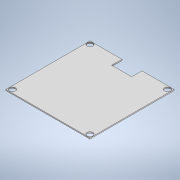
# Autodesk Inventor part: Bottom Cover
Saved by Autodesk Inventor 2020 (Build 240168000, 168)
## iProperties
Created: 2019-07-24
Part Number: Bottom Cover
Material: Generic
Document SubType Name: Modeling
Designer: Paul
Density: 1 g/cm^3
Appearance: Default
Author: Paul
Autodesk Inventor part; units mm, degrees
ref_plane "YZ Plane" through (0, 0, 0) normal (1, 0, 0) x (0, 1, 0)
ref_plane "XZ Plane" through (0, 0, 0) normal (0, 1, 0) x (-1, 0, 0)
ref_plane "XY Plane" through (0, 0, 0) normal (0, 0, 1) x (1, 0, 0)
sketch "Sketch1" plane through (0, 0, 0) normal (0, 1, 0) x (-1, 0, 0)
  line L0 (16, 16) -> (-16, 16)
  line L1 (-16, 16) -> (-16, -16)
  line L2 (-16, -16) -> (16, -16)
  line L3 (16, -16) -> (16, 16)
  line L4 (16, 16) -> (-16, -16) construction
  line L5 (-16, 16) -> (16, -16) construction
  point P0 (0, 0)
  dimension "d0" = 32
  dimension "d1" = 32
  constraints: 12 end point, 2 midpoint, 2 parallel, 1 horizontal, 1 perpendicular
  measures "d0" distance of L2.end L1.end
  measures "d1" distance of L1.end L0.end
extrude "Extrusion1" add sketch "Sketch1" along normal blind 0.4
sketch "Sketch2" plane through (0, 0.4, 0) normal (0, 1, 0) x (1, 0, 0)
  circle A0 centre (-14.76, -14.76) radius 1.11
  circle A1 centre (-14.76, 14.76) radius 1.11
  circle A2 centre (14.76, 14.76) radius 1.11
  circle A3 centre (14.76, -14.76) radius 1.11
  line L0 (16, 16) -> (-16, 16) projected
  line L1 (-16, 16) -> (-16, -16) projected
  line L2 (16, -16) -> (16, 16) projected
  line L3 (-16, -16) -> (16, -16) projected
  point P0 (0, 0)
  dimension "d16" = 2.22
  dimension "d17" = 2.22
  dimension "d18" = 2.22
  dimension "d19" = 2.22
  dimension "d20" = 1.24
  dimension "d21" = 1.24
  dimension "d22" = 1.24
  dimension "d23" = 1.24
  dimension "d24" = 1.24
  dimension "d25" = 1.24
  dimension "d26" = 1.24
  dimension "d27" = 1.24
  constraints: 4 centre point
  measures "d16" diameter of A0
  measures "d17" diameter of A1
  measures "d18" diameter of A2
  measures "d19" diameter of A3
  measures "d20" distance from line of L0 A1.centre
  measures "d21" distance from line of L1 A1.centre
  measures "d22" distance from line of L0 A2.centre
  measures "d23" distance from line of L2 A2.centre
  measures "d24" distance from line of L2 A3.centre
  measures "d25" distance from line of L3 A3.centre
  measures "d26" distance from line of L1 A0.centre
  measures "d27" distance from line of L3 A0.centre
extrude "Extrusion2" cut sketch "Sketch2" against normal blind 0.4 contours A0 | A1 | A2 | A3
sketch "Sketch3" plane through (0, 0.4, 0) normal (0, 1, 0) x (1, 0, 0)
  line L0 (-3.8, 16) -> (3.8, 16)
  line L1 (3.8, 16) -> (3.8, 12.1)
  line L2 (3.8, 12.1) -> (-3.8, 12.1)
  line L3 (-3.8, 12.1) -> (-3.8, 16)
  line L4 (16, 16) -> (-16, 16) projected
  line L5 (16, -16) -> (16, 16) projected
  dimension "d32" = 7.6
  dimension "d33" = 3.9
  dimension "d34" = 0
  dimension "d35" = 12.2
  constraints: 8 end point, 2 parallel, 1 horizontal, 1 perpendicular
  measures "d32" distance of L1.end L2.end
  measures "d33" distance of L0.end L1.end
  measures "d34" distance between parallel lines of L4 L0
  measures "d35" distance between parallel lines of L5 L1
extrude "Extrusion3" cut sketch "Sketch3" against normal blind 0.4
body "Solid1"
